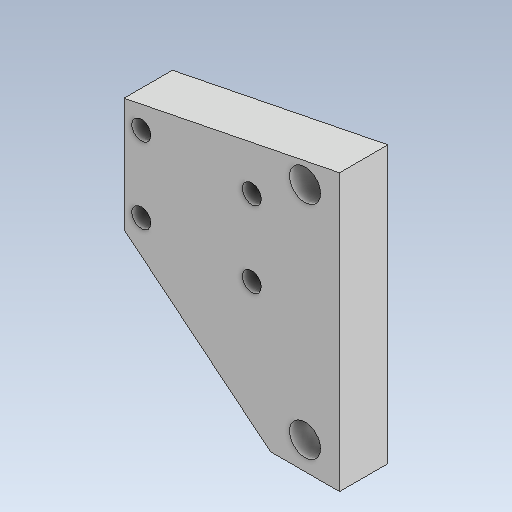
# Autodesk Inventor part: Part21
Saved by Autodesk Inventor 2020.2 (Build 242310000, 310)
## iProperties
Created: 2022-11-16
Part Number: Part21
Material: 一般
Document SubType Name: Modeling
Designer: Administrator
Density: 1 g/cm^3
Appearance: 既定
Author: Administrator
Autodesk Inventor part; units mm, degrees
ref_plane "YZ Plane" through (0, 0, 0) normal (1, 0, 0) x (0, 1, 0)
ref_plane "XZ Plane" through (0, 0, 0) normal (0, 1, 0) x (-1, 0, 0)
ref_plane "XY Plane" through (0, 0, 0) normal (0, 0, 1) x (1, 0, 0)
sketch "スケッチ1 outline for 押し出し1" plane through (0, 0, 0) normal (0, 0, 1) x (1, 0, 0)
  line L0 (-1089.396157, 354.695803) -> (-1151.82556, 342.195803)
  line L1 (-1089.396157, 274.695803) -> (-1089.396157, 354.695803)
  line L2 (-1151.82556, 342.195803) -> (-1151.82556, 309.195803)
  line L3 (-1109.396157, 274.695803) -> (-1089.396157, 274.695803)
  line L4 (-1151.82556, 309.195803) -> (-1109.396157, 274.695803)
  circle A0 centre (-1099.396157, 282.695803) radius 4.5
  circle A1 centre (-1146.82556, 314.695803) radius 2.75
  circle A2 centre (-1146.82556, 336.695803) radius 2.75
  circle A3 centre (-1114.82556, 314.695803) radius 2.75
  circle A4 centre (-1114.82556, 336.695803) radius 2.75
  circle A5 centre (-1099.396157, 346.695803) radius 4.5
extrude "押し出し1" add sketch "スケッチ1 outline for 押し出し1" along normal blind 14.016552
